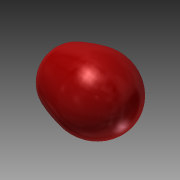
# Autodesk Inventor part: tool_3
Saved by Autodesk Inventor 2015 (Build 190159000, 159)
## iProperties
Created: 2015-12-22
Part Number: tool_3
Material: ゴム、シリコーン
Document SubType Name: Modeling
Designer: Ryo
Density: 1.25 g/cm^3
Appearance: ゴム - 黒 - バージョン 1.1
Author: Ryo
Autodesk Inventor part; units mm, degrees
ref_plane "YZ Plane" through (0, 0, 0) normal (1, 0, 0) x (0, 1, 0)
ref_plane "XZ Plane" through (0, 0, 0) normal (0, 1, 0) x (-1, 0, 0)
ref_plane "XY Plane" through (0, 0, 0) normal (0, 0, 1) x (1, 0, 0)
sketch "スケッチ1" plane through (0, 0, 0) normal (0, 1, 0) x (-1, 0, 0)
  line L0 (22.9969, 0) -> (-57.0031, 0)
  arc A0 (6.4278, -25.7197) -> (22.9969, 0) centre (-3.101, -1.3841) ccw
  arc A1 (-15.0762, -31.9762) -> (6.4278, -25.7197) centre (-38.9589, 90.1932) ccw
  arc A2 (-49.682, -20.2968) -> (-15.0762, -31.9762) centre (-22.1454, 4.1857) ccw
  arc A3 (-57.0031, 0) -> (-49.682, -20.2968) centre (-27.9768, -0.9989) ccw
  point P0 (0, 0)
  dimension "d0" = 80
  constraints: 8 point on circle, 4 centre point, 3 tangent, 2 end point, 1 horizontal
  measures "d0" distance of L0.start L0.end
revolve "回転1" add sketch "スケッチ1" angle 360 about axis through (-22.9969, 0, 0) along (1, 0, 0)
